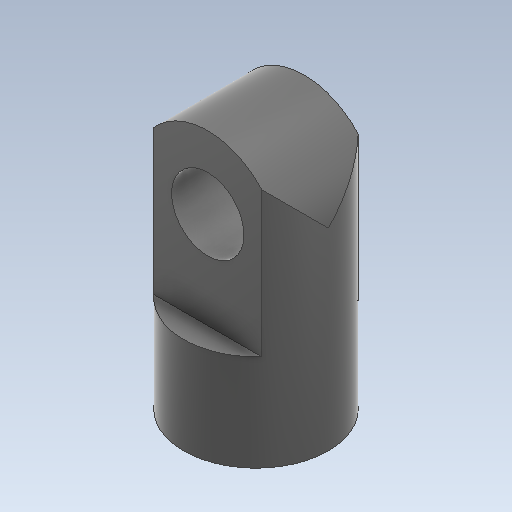
# Autodesk Inventor part: 頭
Saved by Autodesk Inventor 2020 (Build 240168000, 168)
## iProperties
Created: 2020-03-29
Part Number: 頭
Material: ABS プラスチック
Document SubType Name: Modeling
Designer: happy
Density: 1.06 g/cm^3
Appearance: 滑らか - 黒
Mass: 0.288187 g
Surface Area: 3.02239 cm^2
Volume: 0.271875 cm^3
Author: happy
Autodesk Inventor part; units mm, degrees
ref_plane "YZ Plane" through (0, 0, 0) normal (1, 0, 0) x (0, 1, 0)
ref_plane "XZ Plane" through (0, 0, 0) normal (0, 1, 0) x (-1, 0, 0)
ref_plane "XY Plane" through (0, 0, 0) normal (0, 0, 1) x (1, 0, 0)
sketch "スケッチ3" plane through (0, 0, 0) normal (0, 0, 1) x (1, 0, 0)
  circle A0 centre (0, 0) radius 1.5
  circle A1 centre (0, 0) radius 3
  line L0 (3, 0) -> (3, -4)
  line L1 (3, -4) -> (-3, -4)
  line L2 (-3, -4) -> (-3, 0)
  dimension "d9" = 6
  dimension "d8" = 3
  dimension "d10" = 4
  constraints: 6 end point, 3 vertical, 2 coincident, 1 centre point, 1 parallel, 3 other
  measures "d8" diameter of A0
  measures "d10" distance from line of L1 A0.centre
extrude "押し出し3" add sketch "スケッチ3" along normal blind 4
sketch "スケッチ4" plane through (-3, -4, 0) normal (0, -1, 0) x (1, 0, 0)
  line L0 (6, 4) -> (0, 4) projected
  line L1 (6, 0) -> (6, 4) projected
  circle A0 centre (3, 2) radius 3
  line L2 (0, 0) -> (0, 4) projected
  line L3 (4.0287, 2) -> (1.8756, 2)
  point P0 (3, 0)
  point P1 (6, 2)
  constraints: 2 end point, 2 tangent, 1 centre point, 1 horizontal, 1 midpoint, 1 point on line
extrude "押し出し4" cut sketch "スケッチ4" against normal blind 10 contours A0 L0 | L0 A0 keep common part
extrude "押し出し5" add sketch "スケッチ4" along normal blind 4 contours A0 L0 | L0 A0
